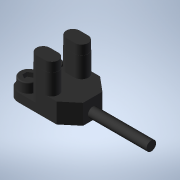
# Autodesk Inventor part: ETH2-14-sensor
Saved by Autodesk Inventor 2021 (Build 250183000, 183)
## iProperties
Created: 2025-05-01
Part Number: ETH2-14-sensor
Material: Generic
Catalog Web Link: www.cadenas.de
Description: GTH4 SENSOR-GTH4 Sensor
Vendor: TOYO
Document SubType Name: Modeling
Designer: psAdmin
Manufacturer: TOYO
Mass: 1.95317 g
Surface Area: 14.6479 cm^2
Volume: 1.95317 cm^3
Density: 1 g/cm^3
Appearance: PSOLRGB-175-175-175
Category: PARTsolutions
Company: TOYO
Title: ETH2-14-sensor
Author: Cadenas PARTsolutions
Comments: GTH4 Sensor
PSOL_IDENT_0: {$CADENAS_DATA/23d-libs/toyo/eth2_series/sensor/gth4_sensor.prj},173 {VTYP=3D},{NB=ETH2-14-sensor},{
PSOL_IDENT_1: LINA=ETH2-14-sensor},{NN=GTH4 SENSOR},{DATE=02.07.2024 05:59:00},{GEOMDATE=27.06.2024 08:07:24},{VER
PSOL_IDENT_2: SION=},{LINEID=10},{WBVAR=},{WBNUMERIC=}  {NB=ETH2-14-sensor},{LINA=ETH2-14-sensor},{KT=DUMMY},{IDNR=
PSOL_IDENT_3: },{MODEL=ETH2-14}
NB: ETH2-14-sensor
NN: GTH4 SENSOR
NT: GTH4 Sensor
NBSYN: $MODEL.-sensor
LINA: ETH2-14-sensor
CATALOG: TOYO
MODEL: ETH2-14
SUPPLIER: TOYO
ARTICLENO: ETH2-14-sensor
BOMINFO: ETH2-14-sensor
CREATOR: CADENAS GmbH
Autodesk Inventor part; units mm, degrees
sketch "Sketch_1" plane through (0, 0, 0) normal (0, 0, 1) x (1, 0, 0)
  line L0 (0, 2.6) -> (0, 0)
  line L1 (0, 0) -> (20, 0)
  line L2 (20, 0) -> (20, 6.2)
  line L3 (20, 6.2) -> (7, 6.2)
  line L4 (7, 6.2) -> (7, 2.6)
  line L5 (7, 2.6) -> (0, 2.6)
  constraints: 12 end point
extrude "Extrusion1" add sketch "Sketch_1" along normal mid plane 13.6
fillet "Fillet1" radius 3.5 2 edges at (0, 1.3, 6.8) (0, 1.3, -6.8)
fillet "Fillet2" radius 2.15 2 edges at (7, 4.4, 6.8) (7, 4.4, -6.8)
sketch "Sketch_4" plane through (20, 0, 0) normal (1, 0, 0) x (0, 0, -1)
  circle A0 centre (0, 2.2) radius 1.5
  constraints: 1 centre point
extrude "Extrusion2" add sketch "Sketch_4" along normal blind 18.3
sketch "Sketch_7" plane through (0, 0, 3.5) normal (0, 0, 1) x (1, 0, 0)
  line L0 (3.5, 2.6) -> (3.5, 5.6)
  line L1 (3.5, 5.6) -> (5.95, 5.6)
  arc A0 (6.25, 5.3) -> (5.95, 5.6) centre (5.95, 5.3) ccw
  line L2 (6.25, 5.3) -> (6.25, 2.6)
  line L3 (6.25, 2.6) -> (3.5, 2.6)
  line L4 (3.5, 2.6) -> (3.5, 5.6)
  constraints: 10 end point, 2 point on circle, 1 centre point
revolve "Revolution1" add sketch "Sketch_7" angle 360 about axis through (3.5, 2.6, 3.5) along (0, -1, 0)
pattern_linear "Rectangular Pattern1" count 2 spacing 7 along (0, 0, -1) of "Revolution1"
sketch "Sketch_9" plane through (0, 5.6, 0) normal (0, 1, 0) x (1, 0, 0)
  line L0 (2.25, -4.2217) -> (3.5, -4.9434)
  line L1 (3.5, -4.9434) -> (4.75, -4.2217)
  line L2 (4.75, -4.2217) -> (4.75, -2.7783)
  line L3 (4.75, -2.7783) -> (3.5, -2.0566)
  line L4 (3.5, -2.0566) -> (2.25, -2.7783)
  line L5 (2.25, -2.7783) -> (2.25, -4.2217)
  constraints: 12 end point
extrude "Extrusion3" cut sketch "Sketch_9" against normal blind 1.3
pattern_linear "Rectangular Pattern2" count 2 spacing 7 along (0, 0, -1) of "Extrusion3"
sketch "__1" plane through (0, 6.2, 0) normal (0, 1, 0) x (1, 0, 0)
  arc A0 (9.15, -2.5) -> (9.15, -6.8) centre (9.15, -4.65) ccw
  line L0 (9.15, -6.8) -> (11.85, -6.8)
  arc A1 (11.85, -6.8) -> (11.85, -2.5) centre (11.85, -4.65) ccw
  line L1 (11.85, -2.5) -> (9.15, -2.5)
  constraints: 4 end point, 4 point on circle, 2 centre point
extrude "Extrusion4" add sketch "__1" along normal blind 6.4
sketch "__2" plane through (0, 6.2, 0) normal (0, 1, 0) x (1, 0, 0)
  arc A0 (9.15, 6.8) -> (9.15, 2.5) centre (9.15, 4.65) ccw
  line L0 (9.15, 2.5) -> (11.85, 2.5)
  arc A1 (11.85, 2.5) -> (11.85, 6.8) centre (11.85, 4.65) ccw
  line L1 (11.85, 6.8) -> (9.15, 6.8)
  constraints: 4 end point, 4 point on circle, 2 centre point
extrude "Extrusion5" add sketch "__2" along normal blind 6.4
sketch "__3" plane through (0, 12.6, 0) normal (0, 1, 0) x (1, 0, 0)
  arc A0 (9.15, -2.57) -> (9.15, -6.73) centre (9.15, -4.65) ccw
  line L0 (9.15, -6.73) -> (11.85, -6.73)
  arc A1 (11.85, -6.73) -> (11.85, -2.57) centre (11.85, -4.65) ccw
  line L1 (11.85, -2.57) -> (9.15, -2.57)
  constraints: 4 end point, 4 point on circle, 2 centre point
extrude "Extrusion6" add sketch "__3" along normal blind 2.9
sketch "__4" plane through (0, 12.6, 0) normal (0, 1, 0) x (1, 0, 0)
  arc A0 (9.15, 6.73) -> (9.15, 2.57) centre (9.15, 4.65) ccw
  line L0 (9.15, 2.57) -> (11.85, 2.57)
  arc A1 (11.85, 2.57) -> (11.85, 6.73) centre (11.85, 4.65) ccw
  line L1 (11.85, 6.73) -> (9.15, 6.73)
  constraints: 4 end point, 4 point on circle, 2 centre point
extrude "Extrusion7" add sketch "__4" along normal blind 2.9
sketch "__5" plane through (0, 0, 0) normal (0, 1, 0) x (-1, 0, 0)
  line L0 (-15.5, 6.8) -> (-20, 6.8)
  line L1 (-20, 6.8) -> (-20, 3.0241)
  line L2 (-20, 3.0241) -> (-15.5, 6.8)
  constraints: 6 end point
extrude "Extrusion8" cut sketch "__5" along normal blind 10
sketch "__6" plane through (0, 0, 0) normal (0, 1, 0) x (-1, 0, 0)
  line L0 (-15.5, -6.8) -> (-20, -3.0241)
  line L1 (-20, -3.0241) -> (-20, -6.8)
  line L2 (-20, -6.8) -> (-15.5, -6.8)
  constraints: 6 end point
extrude "Extrusion9" cut sketch "__6" along normal blind 10
ref_plane "gth4_sensor_XY" through (0, 0, 0) normal (1, 0, 0) x (0, 0, -1)
ref_plane "gth4_sensor_YZ" through (0, 0, 0) normal (0, 0, -1) x (0, 1, 0)
ref_plane "gth4_sensor_ZX" through (0, 0, 0) normal (0, 1, 0) x (1, 0, 0)
body "Solid1"
